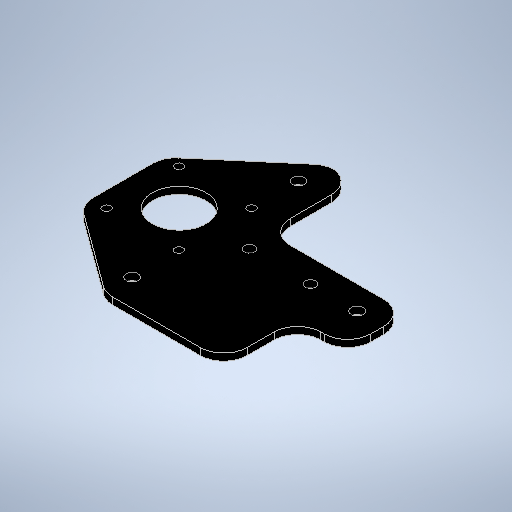
# Autodesk Inventor part: X Motor Bracket
Saved by Autodesk Inventor 2025 (Build 290162000, 162)
## iProperties
Manager: J. Wilburn
Created: 2025-03-12
Part Number: X Motor Bracket
Material: Aluminum 6061
Document SubType Name: Modeling
Designer: MAL16204
Density: 2.7 g/cm^3
Appearance: Anodized - Black
Mass: 46.3508 g
Surface Area: 130.49 cm^2
Volume: 17.1669 cm^3
Author: Richard Malstrom
Title: X Motor Bracket
Subject: Ender 3 Pro Assembly
Autodesk Inventor part; units mm, degrees
ref_plane "YZ Plane" through (0, 0, 0) normal (1, 0, 0) x (0, 1, 0)
ref_plane "XZ Plane" through (0, 0, 0) normal (0, 1, 0) x (-1, 0, 0)
ref_plane "XY Plane" through (0, 0, 0) normal (0, 0, 1) x (1, 0, 0)
sketch "Sketch1" plane through (0, 0, 0) normal (0, 1, 0) x (-1, 0, 0)
  line L0 (-40.9159, 0.459) -> (-78.26, 0.459)
  line L1 (-109.64, -41.041) -> (-109.64, -46.541)
  line L2 (-39.76, -94.041) -> (-41.3348, -94.041)
  line L3 (0, -57.4156) -> (0, -32.0844)
  circle A0 centre (-22.26, -46.541) radius 11.5
  line L4 (-3.5248, -65.0361) -> (-34.8596, -91.6615)
  line L5 (-4.1082, -24.0044) -> (-35.0241, -1.461)
  line L6 (-49.76, -84.041) -> (-49.76, -66.541)
  line L7 (-59.76, -56.541) -> (-99.64, -56.541)
  line L8 (-98.26, -31.041) -> (-99.64, -31.041)
  line L9 (-88.26, -9.541) -> (-88.26, -21.041)
  arc A1 (-3.5248, -65.0361) -> (0, -57.4156) centre (-10, -57.4156) ccw
  arc A2 (0, -32.0844) -> (-4.1082, -24.0044) centre (-10, -32.0844) ccw
  arc A3 (-35.0241, -1.461) -> (-40.9159, 0.459) centre (-40.9159, -9.541) ccw
  arc A4 (-78.26, 0.459) -> (-88.26, -9.541) centre (-78.26, -9.541) ccw
  arc A5 (-98.26, -31.041) -> (-88.26, -21.041) centre (-98.26, -21.041) ccw
  arc A6 (-99.64, -31.041) -> (-109.64, -41.041) centre (-99.64, -41.041) ccw
  arc A7 (-109.64, -46.541) -> (-99.64, -56.541) centre (-99.64, -46.541) ccw
  arc A8 (-49.76, -66.541) -> (-59.76, -56.541) centre (-59.76, -66.541) ccw
  arc A9 (-49.76, -84.041) -> (-39.76, -94.041) centre (-39.76, -84.041) ccw
  arc A10 (-41.3348, -94.041) -> (-34.8596, -91.6615) centre (-41.3348, -84.041) ccw
  point P0 (0, 0)
  point P1 (0, -62.041)
  point P2 (-37.66, -94.041)
  point P3 (0, -27)
  point P4 (-37.6572, 0.459)
  point P5 (0, -44.75)
  point P6 (-40.5474, -94.01)
  dimension "d0" = 94.5
  dimension "d1" = 109.64
  dimension "d2" = 23
  dimension "d3" = 47
  dimension "d4" = 22.26
  dimension "d5" = 37.66
  dimension "d6" = 32
  dimension "d7" = 37.66
  dimension "d8" = 27
  dimension "d11" = 57
  dimension "d12" = 49.76
  dimension "d15" = 25.5
  dimension "d16" = 88.26
  dimension "d17" = 10
  constraints: 20 end point, 20 point on circle, 20 tangent, 11 centre point, 9 equal radius, 8 point on line, 3 parallel, 2 horizontal, 1 midpoint, 1 perpendicular, 1 other
  measures "d0" distance between parallel lines of L2 L0
  measures "d1" distance between parallel lines of L3 L1
  measures "d2" diameter of A0
  measures "d3" distance from line of L0 A0.centre
  measures "d4" distance from line of L3 A0.centre
  measures "d5" distance from line of point (-37.66, -94.041) L3
  measures "d6" distance from line of point (0, -62.041) L2
  measures "d7" distance of point (-37.657, 0.459) point (0, 0)
  measures "d8" distance of point (0, -27) point (0, 0)
  measures "d11" distance between parallel lines of L0 L7
  measures "d12" distance between parallel lines of L3 L6
  measures "d15" distance between parallel lines of L7 L8
  measures "d16" distance between parallel lines of L3 L9
  measures "d17" radius of A1
extrude "Extrusion1" add sketch "Sketch1" along normal blind 3 contours A3 L5 A2 L3 A1 L4 A10 A9 L6 A8 L7 A7 L1 A6 L8 A5 L9 A4 L0
sketch "Sketch2" plane through (0, 3, 0) normal (0, 1, 0) x (1, 0, 0)
  line L0 (40.9159, -0.459) -> (78.26, -0.459) projected
  line L1 (0, 57.4156) -> (0, 32.0844) projected
  point P0 (0, 0)
  point P1 (6.76, 62.041)
  point P2 (37.66, 62.041)
  point P3 (37.66, 31.041)
  point P4 (6.76, 31.041)
  dimension "d20" = 31.5
  dimension "d21" = 37.66
  dimension "d22" = 62.5
  dimension "d23" = 6.76
  constraints: 2 horizontal alignment, 2 vertical alignment
  measures "d20" distance from line of L0 point (6.76, 31.041)
  measures "d21" distance from line of L1 point (37.66, 31.041)
  measures "d22" distance from line of L0 point (6.76, 62.041)
  measures "d23" distance from line of L1 point (6.76, 31.041)
hole "Hole1" at (6.76, 3, -62.041) at (37.66, 3, -62.041) at (37.66, 3, -31.041) at (6.76, 3, -31.041) direction (0, -1, 0) diameter 3.5 end through all
sketch "Sketch3" plane through (0, 3, 0) normal (0, 1, 0) x (1, 0, 0)
  line L0 (40.9159, -0.459) -> (78.26, -0.459) projected
  line L1 (0, 57.4156) -> (0, 32.0844) projected
  point P0 (0, 0)
  point P1 (37.66, 82.041)
  point P2 (37.66, 11.041)
  dimension "d31" = 82.5
  dimension "d32" = 11.5
  dimension "d33" = 37.66
  constraints: 1 vertical alignment
  measures "d31" distance from line of L0 point (37.66, 82.041)
  measures "d32" distance from line of L0 point (37.66, 11.041)
  measures "d33" distance from line of L1 point (37.66, 11.041)
hole "Hole2" at (37.66, 3, -82.041) at (37.66, 3, -11.041) direction (0, -1, 0) diameter 5.1 end through all
sketch "Sketch4" plane through (0, 3, 0) normal (0, 1, 0) x (1, 0, 0)
  line L0 (40.9159, -0.459) -> (78.26, -0.459) projected
  line L1 (0, 57.4156) -> (0, 32.0844) projected
  point P0 (0, 0)
  point P1 (52.26, 46.541)
  point P2 (78.26, 46.541)
  dimension "d41" = 47
  dimension "d42" = 52.26
  dimension "d43" = 78.26
  constraints: 1 horizontal alignment
  measures "d41" distance from line of L0 point (52.26, 46.541)
  measures "d42" distance from line of L1 point (52.26, 46.541)
  measures "d43" distance from line of L1 point (78.26, 46.541)
hole "Hole3" at (52.26, 3, -46.541) at (78.26, 3, -46.541) direction (0, -1, 0) diameter 4.5 end through all
sketch "Sketch5" plane through (0, 3, 0) normal (0, 1, 0) x (1, 0, 0)
  line L0 (0, 57.4156) -> (0, 32.0844) projected
  line L1 (40.9159, -0.459) -> (78.26, -0.459) projected
  point P0 (0, 0)
  point P1 (98.26, 46.541)
  dimension "d51" = 98.26
  dimension "d52" = 47
  measures "d51" distance from line of L0 point (98.26, 46.541)
  measures "d52" distance from line of L1 point (98.26, 46.541)
hole "Hole4" at (98.26, 3, -46.541) direction (0, -1, 0) diameter 5.2 end through all
body "Solid1"
